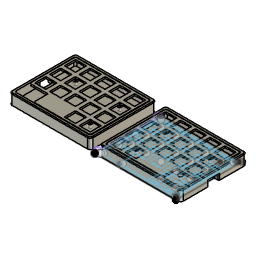
thorium4 (Autodesk Fusion 360 design; units mm, degrees)
Autodesk Fusion 360 part; units mm, degrees
note: some values were not read from the file. Chosen so that the rebuilt part matches the saved one: which bodies a step acts on. Set by a fixed rule: the direction of a hole.
sketch "CaseOuter" plane through (0, 0, 0) normal (0, 0, 1) x (1, 0, 0)
  line L0 (3.5, 0) -> (100.5, 0)
  line L1 (104, 3.5) -> (104, 81.5)
  line L2 (100.5, 85) -> (3.5, 85)
  line L3 (0, 81.5) -> (0, 3.5)
  arc A0 (3.5, 85) -> (0, 81.5) centre (3.5, 81.5) ccw
  arc A1 (104, 81.5) -> (100.5, 85) centre (100.5, 81.5) ccw
  arc A2 (100.5, 0) -> (104, 3.5) centre (100.5, 3.5) ccw
  arc A3 (0, 3.5) -> (3.5, 0) centre (3.5, 3.5) ccw
  point P0 (104, 0)
  point P1 (104, 85)
  point P2 (0, 85)
  dimension "d1" = 104
  dimension "d2" = 85
  dimension "d3" = 104
  dimension "d15" = 3.5
  dimension "d16" = 3.5
  dimension "d17" = 3.5
  dimension "d18" = 3.5
  constraint horizontal L0
  constraint perpendicular L0 L1
  constraint horizontal L2
  constraint coincident P2 L3
  constraint coincident P2 L2
  constraint tangent L3 A0
  constraint tangent L2 A0
  constraint coincident P1 L2
  constraint coincident P1 L1
  constraint tangent L2 A1
  constraint tangent L1 A1
  constraint coincident P0 L1
  constraint coincident P0 L0
  constraint tangent L1 A2
  constraint tangent L0 A2
  constraint coincident origin L0
  constraint tangent L3 A3
  constraint tangent L0 A3
  measures "d1" distance of origin P0
  measures "d2" distance of P0 P1
  measures "d3" distance of P1 P2
  measures "d15" radius of A0
  measures "d16" radius of A1
  measures "d17" radius of A2
  measures "d18" radius of A3
sketch "CaseInner" plane through (0, 0, 0) normal (0, 0, 1) x (1, 0, 0)
  line L0 (5.5, 3.5) -> (98.5, 3.5)
  line L1 (100.5, 5.5) -> (100.5, 79.5)
  line L2 (98.5, 81.5) -> (5.5, 81.5)
  line L3 (3.5, 79.5) -> (3.5, 5.5)
  arc A0 (5.5, 81.5) -> (3.5, 79.5) centre (5.5, 79.5) ccw
  arc A1 (100.5, 79.5) -> (98.5, 81.5) centre (98.5, 79.5) ccw
  arc A2 (98.5, 3.5) -> (100.5, 5.5) centre (98.5, 5.5) ccw
  arc A3 (3.5, 5.5) -> (5.5, 3.5) centre (5.5, 5.5) ccw
  point P0 (3.5, 3.5)
  point P1 (100.5, 3.5)
  point P2 (100.5, 81.5)
  point P3 (3.5, 81.5)
  dimension "d4" = 97
  dimension "d5" = 78
  dimension "d6" = 97
  dimension "d19" = 2
  constraint horizontal L0
  constraint vertical L1
  constraint horizontal L2
  constraint coincident P3 L2
  constraint coincident P3 L3
  constraint tangent L2 A0
  constraint tangent L3 A0
  constraint coincident P2 L2
  constraint coincident P2 L1
  constraint tangent L2 A1
  constraint tangent L1 A1
  constraint equal A0 A1
  constraint coincident P1 L1
  constraint coincident P1 L0
  constraint tangent L1 A2
  constraint tangent L0 A2
  constraint equal A0 A2
  constraint coincident P0 L0
  constraint coincident P0 L3
  constraint tangent L0 A3
  constraint tangent L3 A3
  constraint equal A0 A3
  measures "d4" distance of P0 P1
  measures "d5" distance of P1 P2
  measures "d6" distance of P2 P3
  measures "d19" radius of A0
sketch "CaseStandOff" plane through (0, 0, 0) normal (0, 0, 1) x (1, 0, 0)
  circle A0 centre (23.5, 23.5) radius 2.6
  circle A1 centre (23.5, 61.5) radius 2.6
  circle A2 centre (80.5, 61.5) radius 2.6
  circle A3 centre (80.5, 23.5) radius 2.6
  dimension "d11" = 5.2
  dimension "d12" = 5.2
  dimension "d13" = 5.2
  dimension "d14" = 5.2
  measures "d11" diameter of A0
  measures "d12" diameter of A1
  measures "d13" diameter of A2
  measures "d14" diameter of A3
sketch "CaseSwitchHole" plane through (0, 0, 0) normal (0, 0, 1) x (1, 0, 0)
  line L0 (0, 36) -> (5.5, 36)
  line L1 (8, 38.5) -> (8, 46.5)
  line L2 (5.5, 49) -> (0, 49)
  line L3 (0, 49) -> (0, 36)
  arc A0 (8, 46.5) -> (5.5, 49) centre (5.5, 46.5) ccw
  arc A1 (5.5, 36) -> (8, 38.5) centre (5.5, 38.5) ccw
  line L4 (0, 81.5) -> (0, 3.5)
  point P0 (8, 36)
  dimension "d33" = 8
  dimension "d34" = 13
  dimension "d35" = 2.5
  constraint horizontal L0
  constraint vertical L1
  constraint horizontal L2
  constraint vertical L3
  constraint tangent L2 A0
  constraint tangent L1 A0
  constraint coincident P0 L0
  constraint coincident P0 L1
  constraint tangent L0 A1
  constraint tangent L1 A1
  constraint equal A0 A1
  constraint collinear L3 L4
  measures "d33" distance of L0.start P0
  measures "d34" distance of L0.start L2.end
  measures "d35" radius of A0
extrude "Extrude1" add sketch "CaseOuter" along normal blind 13.5 makes body 1
extrude "Extrude2" cut sketch "CaseInner" along normal blind 10 from surface at 3.5 bodies 1
extrude "Extrude9" add sketch "CaseStandOff" along normal blind 4.5 from surface at 2.5 separate body makes body 2 at (80.0485, 58.9395, 4) makes body 3 at (26.0968, 23.3704, 5.5) makes body 4 at (26.0968, 61.3704, 5.5) makes body 5 at (80.4352, 26.0992, 5.5)
hole "Hole1" at (23.5, 61.5, 0) at (80.5, 61.5, 0) at (80.5, 23.5, 0) direction (0, 0, 1) diameter 2.2 depth 10 tip angle 180 countersink diameter 4.4 countersink angle 90 bodies 2 4 5 1
extrude "Extrude4" cut sketch "CaseSwitchHole" along normal blind 8 bodies 1
chamfer "Chamfer1" distance 1 angle 45 8 edges at (0, 42.5, 13.5) (1.0251, 1.0251, 13.5) (52, 0, 13.5) (102.9749, 1.0251, 13.5) (104, 42.5, 13.5) (102.9749, 83.9749, 13.5) (52, 85, 13.5) (1.0251, 83.9749, 13.5) on bodies 1
chamfer "Chamfer2" distance 1 angle 45 1 edges at (0, 49, 4) on bodies 1
chamfer "Chamfer3" distance 1 angle 45 1 edges at (0, 36, 4) on bodies 1
sketch "PlateOuter" plane through (0, 0, 0) normal (0, 0, 1) x (1, 0, 0)
  line L0 (6, 81) -> (98, 81)
  line L1 (100, 79) -> (100, 6)
  line L2 (98, 4) -> (29.5, 4)
  line L3 (27.5, 6) -> (27.5, 22.28)
  line L4 (27.5, 22.28) -> (6, 22.28)
  line L5 (4, 24.28) -> (4, 79)
  arc A0 (6, 81) -> (4, 79) centre (6, 79) ccw
  arc A1 (100, 79) -> (98, 81) centre (98, 79) ccw
  arc A2 (98, 4) -> (100, 6) centre (98, 6) ccw
  arc A3 (27.5, 6) -> (29.5, 4) centre (29.5, 6) ccw
  arc A4 (4, 24.28) -> (6, 22.28) centre (6, 24.28) ccw
  point P0 (4, 4)
  point P1 (100, 4)
  point P2 (4, 81)
  point P3 (100, 4)
  point P4 (27.5, 4)
  point P5 (4, 22.28)
  dimension "d41" = 96
  dimension "d42" = 77
  dimension "d57" = 90
  dimension "d58" = 72.5
  dimension "d59" = 18.28
  dimension "d60" = 23.5
  dimension "d61" = 2
  dimension "d62" = 2
  constraint horizontal L0
  constraint coincident P3 P1
  constraint vertical L3
  constraint perpendicular L0 L5
  constraint tangent L0 A0
  constraint tangent L5 A0
  constraint tangent L0 A1
  constraint tangent L1 A1
  constraint equal A0 A1
  constraint coincident P3 L2
  constraint tangent L1 A2
  constraint tangent L2 A2
  constraint coincident P4 L3
  constraint coincident P4 L2
  constraint tangent L3 A3
  constraint tangent L2 A3
  constraint equal A2 A3
  constraint coincident P5 L5
  constraint coincident P5 L4
  constraint tangent L5 A4
  constraint tangent L4 A4
  constraint equal A2 A4
  measures "d41" distance of P0 P3
  measures "d42" distance of P0 P2
  measures "d57" angle of L1 L2
  measures "d58" distance of P3 P4
  measures "d59" distance of P4 L3.end
  measures "d60" distance of L3.end P5
  measures "d61" radius of A0
  measures "d62" radius of A2
sketch "PlateHole" plane through (0, 0, 0) normal (0, 0, 1) x (1, 0, 0)
  line L0 (97.05, 63.95) -> (82.95, 63.95)
  line L1 (82.95, 63.95) -> (82.95, 78.05)
  line L2 (82.95, 78.05) -> (97.05, 78.05)
  line L3 (97.05, 78.05) -> (97.05, 63.95)
  line L4 (97.05, 63.95) -> (82.95, 78.05) construction
  line L5 (82.95, 63.95) -> (97.05, 78.05) construction
  line L6 (63.95, 78.05) -> (78.05, 78.05)
  line L7 (78.05, 63.95) -> (63.95, 63.95)
  line L8 (78.05, 78.05) -> (78.05, 63.95)
  line L9 (78.05, 63.95) -> (63.95, 78.05) construction
  line L10 (63.95, 63.95) -> (63.95, 78.05)
  line L11 (63.95, 63.95) -> (78.05, 78.05) construction
  line L12 (44.95, 78.05) -> (59.05, 78.05)
  line L13 (59.05, 63.95) -> (44.95, 63.95)
  line L14 (59.05, 78.05) -> (59.05, 63.95)
  line L15 (59.05, 63.95) -> (44.95, 78.05) construction
  line L16 (44.95, 63.95) -> (44.95, 78.05)
  line L17 (44.95, 63.95) -> (59.05, 78.05) construction
  line L18 (25.95, 78.05) -> (40.05, 78.05)
  line L19 (40.05, 63.95) -> (25.95, 63.95)
  line L20 (40.05, 78.05) -> (40.05, 63.95)
  line L21 (40.05, 63.95) -> (25.95, 78.05) construction
  line L22 (25.95, 63.95) -> (25.95, 78.05)
  line L23 (25.95, 63.95) -> (40.05, 78.05) construction
  line L24 (6.95, 78.05) -> (21.05, 78.05)
  line L25 (21.05, 63.95) -> (6.95, 63.95)
  line L26 (21.05, 78.05) -> (21.05, 63.95)
  line L27 (21.05, 63.95) -> (6.95, 78.05) construction
  line L28 (6.95, 63.95) -> (6.95, 78.05)
  line L29 (6.95, 63.95) -> (21.05, 78.05) construction
  line L30 (82.95, 59.05) -> (97.05, 59.05)
  line L31 (97.05, 44.95) -> (82.95, 44.95)
  line L32 (97.05, 59.05) -> (97.05, 44.95)
  line L33 (97.05, 44.95) -> (82.95, 59.05) construction
  line L34 (82.95, 44.95) -> (82.95, 59.05)
  line L35 (82.95, 44.95) -> (97.05, 59.05) construction
  line L36 (63.95, 59.05) -> (78.05, 59.05)
  line L37 (78.05, 44.95) -> (63.95, 44.95)
  line L38 (78.05, 59.05) -> (78.05, 44.95)
  line L39 (78.05, 44.95) -> (63.95, 59.05) construction
  line L40 (63.95, 44.95) -> (63.95, 59.05)
  line L41 (63.95, 44.95) -> (78.05, 59.05) construction
  line L42 (44.95, 59.05) -> (59.05, 59.05)
  line L43 (59.05, 44.95) -> (44.95, 44.95)
  line L44 (59.05, 59.05) -> (59.05, 44.95)
  line L45 (59.05, 44.95) -> (44.95, 59.05) construction
  line L46 (44.95, 44.95) -> (44.95, 59.05)
  line L47 (44.95, 44.95) -> (59.05, 59.05) construction
  line L48 (25.95, 59.05) -> (40.05, 59.05)
  line L49 (40.05, 44.95) -> (25.95, 44.95)
  line L50 (40.05, 59.05) -> (40.05, 44.95)
  line L51 (40.05, 44.95) -> (25.95, 59.05) construction
  line L52 (25.95, 44.95) -> (25.95, 59.05)
  line L53 (25.95, 44.95) -> (40.05, 59.05) construction
  line L54 (6.95, 59.05) -> (21.05, 59.05)
  line L55 (21.05, 44.95) -> (6.95, 44.95)
  line L56 (21.05, 59.05) -> (21.05, 44.95)
  line L57 (21.05, 44.95) -> (6.95, 59.05) construction
  line L58 (6.95, 44.95) -> (6.95, 59.05)
  line L59 (6.95, 44.95) -> (21.05, 59.05) construction
  line L60 (82.95, 40.05) -> (97.05, 40.05)
  line L61 (97.05, 25.95) -> (82.95, 25.95)
  line L62 (97.05, 40.05) -> (97.05, 25.95)
  line L63 (97.05, 25.95) -> (82.95, 40.05) construction
  line L64 (82.95, 25.95) -> (82.95, 40.05)
  line L65 (82.95, 25.95) -> (97.05, 40.05) construction
  line L66 (63.95, 40.05) -> (78.05, 40.05)
  line L67 (78.05, 25.95) -> (63.95, 25.95)
  line L68 (78.05, 40.05) -> (78.05, 25.95)
  line L69 (78.05, 25.95) -> (63.95, 40.05) construction
  line L70 (63.95, 25.95) -> (63.95, 40.05)
  line L71 (63.95, 25.95) -> (78.05, 40.05) construction
  line L72 (44.95, 40.05) -> (59.05, 40.05)
  line L73 (59.05, 25.95) -> (44.95, 25.95)
  line L74 (59.05, 40.05) -> (59.05, 25.95)
  line L75 (59.05, 25.95) -> (44.95, 40.05) construction
  line L76 (44.95, 25.95) -> (44.95, 40.05)
  line L77 (44.95, 25.95) -> (59.05, 40.05) construction
  line L78 (25.95, 40.05) -> (40.05, 40.05)
  line L79 (40.05, 25.95) -> (25.95, 25.95)
  line L80 (40.05, 40.05) -> (40.05, 25.95)
  line L81 (40.05, 25.95) -> (25.95, 40.05) construction
  line L82 (25.95, 25.95) -> (25.95, 40.05)
  line L83 (25.95, 25.95) -> (40.05, 40.05) construction
  line L84 (6.95, 40.05) -> (21.05, 40.05)
  line L85 (21.05, 25.95) -> (6.95, 25.95)
  line L86 (21.05, 40.05) -> (21.05, 25.95)
  line L87 (21.05, 25.95) -> (6.95, 40.05) construction
  line L88 (6.95, 25.95) -> (6.95, 40.05)
  line L89 (6.95, 25.95) -> (21.05, 40.05) construction
  line L90 (82.95, 21.05) -> (97.05, 21.05)
  line L91 (97.05, 6.95) -> (82.95, 6.95)
  line L92 (97.05, 21.05) -> (97.05, 6.95)
  line L93 (97.05, 6.95) -> (82.95, 21.05) construction
  line L94 (82.95, 6.95) -> (82.95, 21.05)
  line L95 (82.95, 6.95) -> (97.05, 21.05) construction
  line L96 (63.95, 21.05) -> (78.05, 21.05)
  line L97 (78.05, 6.95) -> (63.95, 6.95)
  line L98 (78.05, 21.05) -> (78.05, 6.95)
  line L99 (78.05, 6.95) -> (63.95, 21.05) construction
  line L100 (63.95, 6.95) -> (63.95, 21.05)
  line L101 (63.95, 6.95) -> (78.05, 21.05) construction
  point P0 (90, 71)
  point P1 (71, 71)
  point P2 (52, 71)
  point P3 (33, 71)
  point P4 (14, 71)
  point P5 (90, 52)
  point P6 (71, 52)
  point P7 (52, 52)
  point P8 (33, 52)
  point P9 (14, 52)
  point P10 (90, 33)
  point P11 (71, 33)
  point P12 (52, 33)
  point P13 (33, 33)
  point P14 (14, 33)
  point P15 (90, 14)
  point P16 (71, 14)
  dimension "d44" = 14.1
  dimension "d45" = 14.1
  dimension "d53" = -19
  dimension "d54" = -19
  constraint horizontal L0
  constraint perpendicular L0 L1
  constraint parallel L0 L2
  constraint parallel L1 L3
  constraint coincident L4 P0
  constraint coincident L5 P0
  measures "d44" distance of L1.end L2.end
  measures "d45" distance of L0.end L1.end
sketch "PlateHole2" plane through (0, 0, 0) normal (0, 0, 1) x (1, 0, 0)
  line L0 (93, 63.5) -> (87, 63.5)
  line L1 (87, 63.5) -> (87, 78.5)
  line L2 (87, 78.5) -> (93, 78.5)
  line L3 (93, 78.5) -> (93, 63.5)
  line L4 (93, 63.5) -> (87, 78.5) construction
  line L5 (87, 63.5) -> (93, 78.5) construction
  line L6 (68, 63.5) -> (68, 78.5)
  line L7 (68, 78.5) -> (74, 78.5)
  line L8 (74, 78.5) -> (74, 63.5)
  line L9 (74, 63.5) -> (68, 63.5)
  line L10 (49, 63.5) -> (49, 78.5)
  line L11 (49, 78.5) -> (55, 78.5)
  line L12 (55, 78.5) -> (55, 63.5)
  line L13 (55, 63.5) -> (49, 63.5)
  line L14 (30, 63.5) -> (30, 78.5)
  line L15 (30, 78.5) -> (36, 78.5)
  line L16 (36, 78.5) -> (36, 63.5)
  line L17 (36, 63.5) -> (30, 63.5)
  line L18 (11, 63.5) -> (11, 78.5)
  line L19 (11, 78.5) -> (17, 78.5)
  line L20 (17, 78.5) -> (17, 63.5)
  line L21 (17, 63.5) -> (11, 63.5)
  line L22 (87, 44.5) -> (87, 59.5)
  line L23 (87, 59.5) -> (93, 59.5)
  line L24 (93, 59.5) -> (93, 44.5)
  line L25 (93, 44.5) -> (87, 44.5)
  line L26 (68, 44.5) -> (68, 59.5)
  line L27 (68, 59.5) -> (74, 59.5)
  line L28 (74, 59.5) -> (74, 44.5)
  line L29 (74, 44.5) -> (68, 44.5)
  line L30 (49, 44.5) -> (49, 59.5)
  line L31 (49, 59.5) -> (55, 59.5)
  line L32 (55, 59.5) -> (55, 44.5)
  line L33 (55, 44.5) -> (49, 44.5)
  line L34 (30, 44.5) -> (30, 59.5)
  line L35 (30, 59.5) -> (36, 59.5)
  line L36 (36, 59.5) -> (36, 44.5)
  line L37 (36, 44.5) -> (30, 44.5)
  line L38 (11, 44.5) -> (11, 59.5)
  line L39 (11, 59.5) -> (17, 59.5)
  line L40 (17, 59.5) -> (17, 44.5)
  line L41 (17, 44.5) -> (11, 44.5)
  line L42 (87, 25.5) -> (87, 40.5)
  line L43 (87, 40.5) -> (93, 40.5)
  line L44 (93, 40.5) -> (93, 25.5)
  line L45 (93, 25.5) -> (87, 25.5)
  line L46 (68, 25.5) -> (68, 40.5)
  line L47 (68, 40.5) -> (74, 40.5)
  line L48 (74, 40.5) -> (74, 25.5)
  line L49 (74, 25.5) -> (68, 25.5)
  line L50 (49, 25.5) -> (49, 40.5)
  line L51 (49, 40.5) -> (55, 40.5)
  line L52 (55, 40.5) -> (55, 25.5)
  line L53 (55, 25.5) -> (49, 25.5)
  line L54 (30, 25.5) -> (30, 40.5)
  line L55 (30, 40.5) -> (36, 40.5)
  line L56 (36, 40.5) -> (36, 25.5)
  line L57 (36, 25.5) -> (30, 25.5)
  line L58 (11, 25.5) -> (11, 40.5)
  line L59 (11, 40.5) -> (17, 40.5)
  line L60 (17, 40.5) -> (17, 25.5)
  line L61 (17, 25.5) -> (11, 25.5)
  line L62 (87, 6.5) -> (87, 21.5)
  line L63 (87, 21.5) -> (93, 21.5)
  line L64 (93, 21.5) -> (93, 6.5)
  line L65 (93, 6.5) -> (87, 6.5)
  line L66 (68, 6.5) -> (68, 21.5)
  line L67 (68, 21.5) -> (74, 21.5)
  line L68 (74, 21.5) -> (74, 6.5)
  line L69 (74, 6.5) -> (68, 6.5)
  point P0 (90, 71)
  dimension "d72" = 15
  dimension "d75" = -19
  dimension "d76" = -19
  constraint horizontal L0
  constraint perpendicular L0 L1
  constraint parallel L0 L2
  constraint parallel L1 L3
  constraint coincident L4 P0
  constraint coincident L5 P0
  measures "d72" distance of L0.end L1.end
extrude "Extrude5" add sketch "PlateOuter" along normal blind 2.2 from surface at 11.5 separate body makes body 6
extrude "Extrude6" cut sketch "PlateHole" along normal blind 2.2 from surface at 11.5 bodies 6
extrude "Extrude8" cut sketch "PlateHole2" along normal blind 0.7 from surface at 11.5 bodies 6
move_body "Move3" bodies 6 5 2 1 4 3 to x (1, 0, 0) y (0, 1, 0) z (0, 0, 1) at (-110, 0, 0)
mirror "Mirror1" about plane through (0, 0, 0) normal (1, 0, 0) of bodies 6 2 4 1 3 5 makes body 7 at (80.1806, 20.053, 0) makes body 8 at (63.8667, 12.3, 13.7) makes body 9 at (26.9032, 61.3704, 5.5) makes body 10 at (87.3281, 25.9646, 5.5) makes body 11 at (86.5648, 64.0992, 5.5) makes body 12 at (26.9032, 23.3704, 5.5)
copy_body "Body->Comp11" bodies 6 removing the originals makes body 13 in component "PlateL"
copy_body "Body->Comp12" bodies 1 removing the originals makes body 14 in component "CaseL"
copy_body "CutPasteBodies1" bodies 5 2 4 3 removing the originals makes body 15 makes body 16 makes body 17 makes body 18 in component "CaseL"
copy_body "Body->Comp13" bodies 8 removing the originals makes body 19 in component "PlateR"
copy_body "Body->Comp14" bodies 7 removing the originals makes body 20 in component "CaseR"
copy_body "CutPasteBodies1'" bodies 9 10 11 12 removing the originals makes body 21 makes body 22 makes body 23 makes body 24 in component "CaseR"
component "PlateL" placed x (1, 0, 0) y (0, 1, 0) z (0, 0, 1) at (0, 0, 0)
component "CaseL" placed x (1, 0, 0) y (0, 1, 0) z (0, 0, 1) at (0, 0, 0)
component "PlateR" placed x (1, 0, 0) y (0, 1, 0) z (0, 0, 1) at (0, 0, 0)
component "CaseR" placed x (1, 0, 0) y (0, 1, 0) z (0, 0, 1) at (0, 0, 0)
equation "d59 = 17.78 mm + 0.5 mm"
named bodies: "Case", "Plate", "StandOff2", "StandOff4", "StandOff1", "StandOff3", "Case (1)", "Plate (1)", "StandOff2 (1)", "StandOff4 (1)", "StandOff1 (1)", "StandOff3 (1)"
